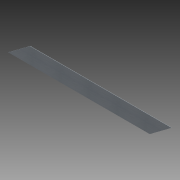
# Autodesk Inventor part: Duct_Outer_Template
Saved by Autodesk Inventor 2011 SP1 (Build 150282100, 282)
## iProperties
Created: 2011-06-12
Part Number: Duct_Outer_Template
Document SubType Name: Modeling
Designer: Andrew G. Meyer
Mass: 80.2386 g
Surface Area: 1035.97 cm^2
Volume: 80.2386 cm^3
Density: 1 g/cm^3
Author: Andrew G. Meyer
Autodesk Inventor part; units mm, degrees
ref_plane "YZ Plane" through (0, 0, 0) normal (1, 0, 0) x (0, 1, 0)
ref_plane "XZ Plane" through (0, 0, 0) normal (0, 1, 0) x (-1, 0, 0)
ref_plane "XY Plane" through (0, 0, 0) normal (0, 0, 1) x (1, 0, 0)
sketch "Sketch1" plane through (0, 0, 0) normal (0, 0, 1) x (1, 0, 0)
  line L0 (-117.1689, -6.1677) -> (-15.5689, 70.0323)
  line L1 (-15.5689, 70.0323) -> (647.7386, 70.0323)
  line L2 (647.7386, 70.0323) -> (546.1386, -6.1677)
  line L3 (546.1386, -6.1677) -> (-117.1689, -6.1677)
  point P0 (0, 0)
  dimension "d0" = 76.2
  dimension "d1" = 663.3075
  dimension "d2" = 101.6
  constraints: 8 end point, 2 parallel, 1 horizontal
  measures "d0" distance between parallel lines of L3 L1
  measures "d1" distance of L0.end L1.end
  measures "d2" horizontal distance of L0.start L0.end
extrude "Extrusion1" add sketch "Sketch1" along normal blind 1.5875
body "Solid1"
